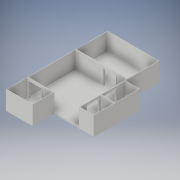
# Autodesk Inventor part: second floor down for landon
Saved by Autodesk Inventor 2017 (Build 210142000, 142)
## iProperties
Created: 2018-05-01
Part Number: second floor down for landon
Material: Generic
Document SubType Name: Modeling
Designer: braxtonwright
Density: 1 g/cm^3
Appearance: Default
Author: braxtonwright
Autodesk Inventor part; units mm, degrees
ref_plane "YZ Plane" through (0, 0, 0) normal (1, 0, 0) x (0, 1, 0)
ref_plane "XZ Plane" through (0, 0, 0) normal (0, 1, 0) x (-1, 0, 0)
ref_plane "XY Plane" through (0, 0, 0) normal (0, 0, 1) x (1, 0, 0)
sketch "Sketch1" plane through (0, 0, 0) normal (0, 1, 0) x (-1, 0, 0)
  line L0 (0, 0) -> (0, -901.7)
  line L1 (0, -901.7) -> (-774.7, -901.7) construction
  line L2 (-393.7, 0) -> (-520.7, 0)
  line L3 (0, 0) -> (0, 317.5)
  line L4 (0, 317.5) -> (-393.7, 317.5)
  line L5 (-393.7, 317.5) -> (-393.7, 0)
  line L6 (0, -901.7) -> (0, -1193.8)
  line L7 (0, -1193.8) -> (-774.7, -1193.8)
  line L8 (-774.7, -317.5) -> (-990.6, -317.5)
  line L9 (-990.6, -317.5) -> (-990.6, 0)
  line L10 (-990.6, 0) -> (-520.7, 0)
  line L11 (-990.6, -317.5) -> (-990.6, -685.8)
  line L12 (-990.6, -685.8) -> (-774.7, -685.8)
  line L13 (-393.7, 0) -> (0, 0) construction
  line L14 (-774.7, -1193.8) -> (-774.7, -901.7)
  line L15 (-774.7, -685.8) -> (-774.7, -901.7)
  dimension "d0" = 901.7
  dimension "d1" = 774.7
  dimension "d2" = 317.5
  dimension "d3" = 393.7
  dimension "d4" = 317.5
  dimension "d5" = 292.1
  dimension "d6" = 317.5
  dimension "d7" = 368.3
  dimension "d9" = 469.9
  dimension "d11" = 990.6
  dimension "d12" = 774.7
  constraints: 32 end point, 5 perpendicular, 4 vertical, 3 horizontal, 1 collinear
  measures "d0" distance of L0.start L0.end
  measures "d1" distance of L0.end L1.end
  measures "d2" distance of L0.start L3.end
  measures "d3" distance of L3.end L4.end
  measures "d4" distance between parallel lines of L2 L4
  measures "d5" distance of L0.end L6.end
  measures "d6" distance between parallel lines of L10 L8
  measures "d7" distance between parallel lines of L12 L8
  measures "d9" distance of L9.end L2.end
  measures "d11" distance between parallel lines of L0 L11
  measures "d12" distance from line of L8.start L0
extrude "floor" add sketch "Sketch1" along normal blind 25.4
sketch "Sketch2" plane through (0, 25.4, 0) normal (0, 1, 0) x (1, 0, 0)
  line L0 (0, 0) -> (0, 719.1204)
  line L1 (0, 719.1204) -> (774.7, 719.1204) construction
  line L2 (0, 0) -> (0, -317.5)
  line L3 (0, -317.5) -> (393.7, -317.5)
  line L4 (393.7, -317.5) -> (393.7, 0)
  line L5 (774.7, 317.5) -> (990.6, 317.5) construction
  line L6 (393.7, 0) -> (0, 0) construction
  line L7 (0, 1193.8) -> (0, -317.5) projected
  line L8 (393.7, 0) -> (990.6, 0) projected
  line L9 (774.7, 719.1204) -> (774.7, 317.5) construction
  line L10 (774.7, 317.5) -> (774.7, 0) construction
  line L11 (387.35, -311.15) -> (6.35, -311.15)
  line L12 (6.35, -311.15) -> (6.35, -6.35)
  line L13 (6.35, -6.35) -> (387.35, -6.35)
  line L14 (387.35, -6.35) -> (387.35, -311.15)
  line L15 (984.25, 679.45) -> (781.05, 679.45)
  line L16 (990.6, 685.8) -> (990.6, 0) projected
  line L17 (990.6, 685.8) -> (774.7, 685.8) projected
  line L18 (520.7, 685.8) -> (520.7, 1193.8) projected
  line L19 (774.7, 1193.8) -> (0, 1193.8) projected
  line L20 (768.35, 0) -> (990.6, 0)
  line L21 (990.6, 0) -> (990.6, 685.8)
  line L22 (990.6, 685.8) -> (774.7, 685.8)
  line L23 (774.7, 685.8) -> (774.7, 1193.8)
  line L24 (774.7, 1193.8) -> (0, 1193.8)
  line L25 (0, 1193.8) -> (0, 719.1204)
  line L26 (781.05, 6.35) -> (984.25, 6.35)
  line L27 (781.05, 311.15) -> (984.25, 311.15)
  line L28 (984.25, 323.85) -> (781.05, 323.85)
  line L29 (781.05, 6.35) -> (781.05, 311.15)
  line L30 (781.05, 323.85) -> (781.05, 679.45)
  line L31 (984.25, 6.35) -> (984.25, 311.15)
  line L32 (984.25, 323.85) -> (984.25, 679.45)
  line L33 (6.35, 6.35) -> (393.7, 6.35)
  line L34 (768.35, 1187.45) -> (6.35, 1187.45)
  line L35 (393.7, 0) -> (393.7, 6.35)
  line L36 (768.35, 6.35) -> (768.35, 0)
  line L37 (6.35, 725.4704) -> (768.35, 725.4704)
  line L38 (768.35, 712.7704) -> (6.35, 712.7704)
  line L39 (768.35, 6.35) -> (768.35, 712.7704)
  line L40 (768.35, 725.4704) -> (768.35, 1187.45)
  line L41 (6.35, 1187.45) -> (6.35, 725.4704)
  line L42 (6.35, 712.7704) -> (6.35, 6.35)
  line L43 (774.7, 685.8) -> (774.7, 1193.8) projected
  line L44 (393.7, -317.5) -> (393.7, 0) projected
  dimension "d27" = 317.5
  dimension "d28" = 6.35
  dimension "d34" = 6.35
  dimension "d39" = 6.35
  dimension "d40" = 6.35
  dimension "d41" = 6.35
  dimension "d42" = 6.35
  dimension "d43" = 6.35
  dimension "d48" = 6.35
  dimension "d50" = 6.35
  dimension "d63" = 12.7
  dimension "d64" = 6.35
  dimension "d67" = 984.25
  dimension "d68" = 0
  dimension "d69" = 679.45
  dimension "d114" = 6.35
  constraints: 74 end point, 14 perpendicular, 11 parallel, 8 collinear, 4 horizontal, 3 vertical, 2 point on line, 3 other
  measures "d27" distance between parallel lines of L5 L8
  measures "d28" distance between parallel lines of L3 L11
  measures "d34" distance between parallel lines of L17 L15
  measures "d39" distance between parallel lines of L26 L8
  measures "d40" distance between parallel lines of L5 L27
  measures "d41" distance between parallel lines of L28 L5
  measures "d42" distance between parallel lines of L16 L31
  measures "d43" horizontal distance of L5.start L27.start
  measures "d48" distance between parallel lines of L33 L8
  measures "d50" distance between parallel lines of L19 L34
  measures "d63" distance between parallel lines of L37 L38
  measures "d64" distance from line of L37.start L1
  measures "d67" distance between parallel lines of L16 L41
  measures "d68" distance from line of L5.end L16
  measures "d69" distance from line of L36.start L17
  measures "d114" distance between parallel lines of L39 L10
extrude "walls" add sketch "Sketch2" along normal blind 254 contours L0 L7 L19 L18 L34 L41 L37 L38 L42 L33 L35 L4 L3 L2 | L19 L23 L17 L16 L8 L36 L39 L38 L18 L37 L40 L34
sketch "Sketch4" plane through (0, 25.4, 0) normal (0, 1, 0) x (1, 0, 0)
  line L0 (387.35, -6.35) -> (6.35, -6.35) projected
  line L1 (387.35, -311.15) -> (387.35, -6.35) projected
  line L2 (6.35, -6.35) -> (387.35, -6.35)
  line L3 (387.35, -6.35) -> (387.35, -311.15)
  line L4 (6.35, -6.35) -> (6.35, -311.15) projected
  line L5 (387.35, -311.15) -> (6.35, -311.15)
  line L6 (6.35, -311.15) -> (6.35, -6.35)
  line L7 (6.35, -311.15) -> (387.35, -311.15) projected
  line L8 (6.35, -311.15) -> (387.35, -311.15)
  line L9 (8.4667, -8.4667) -> (385.2333, -8.4667)
  line L10 (385.2333, -8.4667) -> (385.2333, -309.0333)
  line L11 (385.2333, -309.0333) -> (8.4667, -309.0333)
  line L12 (8.4667, -309.0333) -> (8.4667, -8.4667)
  line L13 (781.05, 311.15) -> (781.05, 6.35) projected
  line L14 (984.25, 6.35) -> (984.25, 311.15) projected
  line L15 (781.05, 311.15) -> (984.25, 311.15)
  line L16 (984.25, 311.15) -> (984.25, 6.35)
  line L17 (984.25, 6.35) -> (781.05, 6.35)
  line L18 (781.05, 6.35) -> (781.05, 311.15)
  line L19 (781.05, 323.85) -> (781.05, 679.45) projected
  line L20 (984.25, 323.85) -> (781.05, 323.85) projected
  line L21 (781.05, 679.45) -> (984.25, 679.45)
  line L22 (984.25, 679.45) -> (984.25, 323.85)
  line L23 (984.25, 323.85) -> (781.05, 323.85)
  line L24 (781.05, 323.85) -> (781.05, 679.45)
  line L25 (982.1333, 677.3333) -> (783.1667, 677.3333)
  line L26 (783.1667, 677.3333) -> (783.1667, 325.9667)
  line L27 (783.1667, 325.9667) -> (982.1333, 325.9667)
  line L28 (982.1333, 325.9667) -> (982.1333, 677.3333)
  line L29 (982.1333, 309.0333) -> (783.1667, 309.0333)
  line L30 (783.1667, 309.0333) -> (783.1667, 8.4667)
  line L31 (783.1667, 8.4667) -> (982.1333, 8.4667)
  line L32 (982.1333, 8.4667) -> (982.1333, 309.0333)
  line L33 (768.35, 725.4704) -> (768.35, 1187.45) projected
  line L34 (768.35, 725.4704) -> (6.35, 725.4704) projected
  line L35 (768.35, 1187.45) -> (6.35, 1187.45)
  line L36 (6.35, 1187.45) -> (6.35, 725.4704)
  line L37 (6.35, 725.4704) -> (768.35, 725.4704)
  line L38 (768.35, 725.4704) -> (768.35, 1187.45)
  line L39 (8.4667, 1185.3333) -> (766.2333, 1185.3333)
  line L40 (766.2333, 1185.3333) -> (766.2333, 727.5871)
  line L41 (766.2333, 727.5871) -> (8.4667, 727.5871)
  line L42 (8.4667, 727.5871) -> (8.4667, 1185.3333)
  line L43 (768.35, 712.7704) -> (768.35, 0) projected
  line L44 (393.7, 6.35) -> (6.35, 6.35) projected
  line L45 (768.35, 712.7704) -> (6.35, 712.7704)
  line L46 (6.35, 712.7704) -> (6.35, 6.35)
  line L47 (768.35, 357.1704) -> (768.35, 712.7704)
  line L48 (766.2333, 710.6538) -> (8.4667, 710.6538)
  line L49 (8.4667, 710.6538) -> (8.4667, 8.4667)
  line L50 (8.4667, 8.4667) -> (395.8167, 8.4667)
  line L51 (766.2333, 359.2871) -> (766.2333, 710.6538)
  line L52 (393.7, 6.35) -> (393.7, 0) projected
  line L53 (393.7, 6.35) -> (393.7, 0)
  line L54 (393.7, 0) -> (395.8167, 0)
  line L55 (990.6, 0) -> (393.7, 0) projected
  line L56 (395.8167, 0) -> (395.8167, 8.4667)
  line L57 (768.35, 357.1704) -> (768.35, 0)
  line L58 (768.35, 0) -> (766.2333, 0)
  line L59 (766.2333, 359.2871) -> (766.2333, 0)
  line L60 (6.35, 6.35) -> (393.7, 6.35)
  line L61 (6.35, 1187.45) -> (768.35, 1187.45) projected
  dimension "d55" = 2.1167
  dimension "d56" = 2.1167
  dimension "d70" = 2.1167
  dimension "d76" = 2.1167
  dimension "d77" = 2.1167
  dimension "d78" = 2.1167
  dimension "d79" = 2.1167
  dimension "d80" = 2.1167
  constraints: 94 end point, 17 parallel, 12 perpendicular, 5 horizontal, 3 collinear, 3 point on line, 13 other
  measures "d55" distance between parallel lines of L21 L25
  measures "d56" distance between parallel lines of L15 L29
  measures "d70" distance between parallel lines of L0 L9
  measures "d76" distance between parallel lines of L35 L39
  measures "d77" distance between parallel lines of L47 L51
  measures "d78" distance of L53.end L54.end
  measures "d79" distance between parallel lines of L44 L50
  measures "d80" distance between parallel lines of L46 L49
extrude "trim" add sketch "Sketch4" along normal blind 21.0312 contours L1 L5 L4 L0 | L15 L14 L17 L13 | L19 L21 L22 L20 | L34 L36 L35 L33 | L43 L55 L59 L51 L48 L49 L50 L56 L54 L52 L44 L46 L45
sketch "Sketch5" plane through (783.1667, 25.4, -8.4667) normal (1, 0, 0) x (0, 0, -1)
  line L0 (0, 0) -> (300.5667, 0) projected
  line L1 (277.2833, 0) -> (86.7833, 0)
  line L2 (86.7833, 0) -> (86.7833, 223.52)
  line L3 (86.7833, 223.52) -> (277.2833, 223.52)
  line L4 (277.2833, 223.52) -> (277.2833, 0)
  line L5 (302.6833, 21.0312) -> (302.6833, 254) projected
  line L6 (315.3833, 21.0312) -> (315.3833, 254) projected
  line L7 (315.3833, 254) -> (302.6833, 254)
  line L8 (-8.4667, 254) -> (677.3333, 254) projected
  line L9 (309.0333, 254) -> (309.0333, -25.4) construction
  line L10 (340.7833, 0) -> (531.2833, 0)
  line L11 (531.2833, 0) -> (531.2833, 223.52)
  line L12 (531.2833, 223.52) -> (340.7833, 223.52)
  line L13 (340.7833, 223.52) -> (340.7833, 0)
  point P0 (-8.4667, -25.4)
  dimension "d59" = 190.5
  dimension "d60" = 223.52
  dimension "d61" = 25.4
  constraints: 20 end point, 4 symmetric about line, 2 parallel, 1 collinear, 1 horizontal, 1 midpoint, 1 perpendicular, 1 point on line, 1 vertical
  measures "d59" distance of L2.end L3.end
  measures "d60" distance of L1.end L2.end
  measures "d61" distance between parallel lines of L5 L4
extrude "doorframe 1 and 2" cut sketch "Sketch5" against normal up to surface (14.8167 mm away)
sketch "Sketch6" plane through (766.2333, 25.4, -727.5871) normal (0, 0, -1) x (-1, 0, 0)
  line L0 (150.2833, 223.52) -> (340.7833, 223.52)
  line L1 (340.7833, 223.52) -> (340.7833, 0)
  line L2 (340.7833, 0) -> (150.2833, 0)
  line L3 (150.2833, 0) -> (150.2833, 223.52)
  line L4 (-8.4667, 7.9325) -> (-8.4667, 240.144)
  line L5 (-8.4667, -25.4) -> (-8.4667, 254) projected
  line L6 (0, 0) -> (757.7667, 0) projected
  point P0 (503.7667, 0)
  point P1 (245.5333, 223.52)
  dimension "d83" = 190.5
  dimension "d84" = 223.52
  dimension "d86" = 254
  constraints: 10 end point, 2 collinear, 2 parallel, 1 horizontal, 1 midpoint, 1 perpendicular, 1 vertical
  measures "d83" distance of L1.end L2.end
  measures "d84" distance of L0.end L1.end
  measures "d86" distance from line of L4 point (245.533, 223.52)
extrude "door frame 3" cut sketch "Sketch6" against normal up to surface (16.9333 mm away)
sketch "Sketch7" plane through (395.8167, 25.4, -8.4667) normal (0, 0, -1) x (-1, 0, 0)
  line L0 (173.5667, 223.52) -> (364.0667, 223.52)
  line L1 (364.0667, 223.52) -> (364.0667, 0)
  line L2 (364.0667, 0) -> (173.5667, 0)
  line L3 (173.5667, 0) -> (173.5667, 223.52)
  line L4 (10.5833, 0) -> (387.35, 0) projected
  line L5 (389.4667, 21.0312) -> (389.4667, 254) projected
  point P0 (395.8167, -25.4)
  dimension "d89" = 190.5
  dimension "d90" = 223.52
  dimension "d91" = 25.4
  constraints: 8 end point, 2 parallel, 1 collinear, 1 horizontal, 1 perpendicular
  measures "d89" distance of L1.end L2.end
  measures "d90" distance of L0.end L1.end
  measures "d91" distance between parallel lines of L5 L1
extrude "door frame 4" cut sketch "Sketch7" against normal up to surface (16.9333 mm away)
ref_plane "door trim workplane 1 and 2" through (774.7, 279.4, -6.35) normal (1, 0, 0) x (0, 0, -1)
sketch "Sketch8" plane through (774.7, 279.4, -6.35) normal (1, 0, 0) x (0, 0, -1)
  line L0 (342.9, -30.48) -> (533.4, -30.48) projected
  line L1 (670.9833, -254) -> (319.6167, -254) projected
  line L2 (533.4, -30.48) -> (342.9, -30.48)
  line L3 (342.9, -30.48) -> (342.9, -254)
  line L4 (533.4, -254) -> (533.4, -30.48)
  line L5 (88.9, -254) -> (88.9, -232.9688) projected
  line L6 (279.4, -30.48) -> (88.9, -30.48)
  line L7 (88.9, -30.48) -> (88.9, -254)
  line L8 (279.4, -254) -> (279.4, -30.48)
  line L9 (541.147, -22.733) -> (335.153, -22.733)
  line L10 (335.153, -22.733) -> (335.153, -254)
  line L11 (541.147, -254) -> (541.147, -22.733)
  line L12 (81.153, -22.733) -> (287.147, -22.733)
  line L13 (287.147, -22.733) -> (287.147, -254)
  line L14 (81.153, -254) -> (81.153, -22.733)
  line L15 (319.6167, -254) -> (670.9833, -254) projected
  line L16 (541.147, -254) -> (533.4, -254)
  line L17 (342.9, -254) -> (335.153, -254)
  line L18 (2.1167, -254) -> (302.6833, -254) projected
  line L19 (287.147, -254) -> (279.4, -254)
  line L20 (88.9, -254) -> (81.153, -254)
  point P0 (-6.35, -279.4)
  dimension "d94" = 7.747
  dimension "d95" = 7.747
  dimension "d96" = 7.747
  dimension "d97" = 7.747
  dimension "d98" = 7.747
  dimension "d99" = 7.747
  constraints: 32 end point, 4 parallel, 4 perpendicular, 4 point on line, 2 collinear, 2 horizontal
  measures "d94" distance between parallel lines of L4 L11
  measures "d95" distance between parallel lines of L6 L12
  measures "d96" distance between parallel lines of L0 L9
  measures "d97" distance between parallel lines of L10 L3
  measures "d98" distance between parallel lines of L8 L13
  measures "d99" distance between parallel lines of L14 L7
extrude "door trim 1 and 2" add sketch "Sketch8" along normal mid plane 25.4 contours L3 L1 L10 L9 L11 L4 L0 | L18 L14 L12 L13 L8 L6 L7 L5
ref_plane "door time workplane 3" through (6.35, 279.4, -719.1204) normal (0, 0, 1) x (1, 0, 0)
sketch "Sketch9" plane through (6.35, 279.4, -719.1204) normal (0, 0, 1) x (1, 0, 0)
  line L0 (609.6, -30.48) -> (419.1, -30.48)
  line L1 (419.1, -30.48) -> (419.1, -254)
  line L2 (609.6, -254) -> (609.6, -30.48)
  line L3 (411.353, -22.733) -> (617.347, -22.733)
  line L4 (617.347, -22.733) -> (617.347, -254)
  line L5 (411.353, -254) -> (411.353, -22.733)
  line L6 (617.347, -254) -> (609.6, -254)
  line L7 (419.1, -254) -> (411.353, -254)
  line L8 (609.6, -232.9688) -> (609.6, -30.48) projected
  line L9 (609.6, -30.48) -> (419.1, -30.48) projected
  line L10 (419.1, -30.48) -> (419.1, -232.9688) projected
  line L11 (759.8833, -254) -> (2.1167, -254) projected
  point P0 (-6.35, -279.4)
  point P1 (-6.35, -279.4)
  dimension "d102" = 7.747
  dimension "d103" = 7.747
  dimension "d104" = 7.747
  constraints: 16 end point, 5 collinear, 3 perpendicular, 2 parallel, 1 horizontal, 1 point on line
  measures "d102" distance between parallel lines of L0 L3
  measures "d103" distance between parallel lines of L2 L4
  measures "d104" distance between parallel lines of L5 L1
extrude "door trim 3" add sketch "Sketch9" along normal mid plane 25.4 contours L0 L1 L7 L5 L3 L4 L6 L2
ref_plane "Work Plane3" through (395.8167, 25.4, 0) normal (0, 0, -1) x (-1, 0, 0)
sketch "Sketch10" plane through (395.8167, 25.4, 0) normal (0, 0, -1) x (-1, 0, 0)
  line L0 (371.8137, 231.267) -> (371.8137, 0)
  line L1 (364.0667, 0) -> (364.0667, 223.52)
  line L2 (371.8137, 0) -> (364.0667, 0)
  line L3 (173.5667, 0) -> (165.8197, 0)
  line L4 (364.0667, 223.52) -> (173.5667, 223.52)
  line L5 (173.5667, 223.52) -> (173.5667, 0)
  line L6 (165.8197, 231.267) -> (371.8137, 231.267)
  line L7 (165.8197, 0) -> (165.8197, 231.267)
  line L8 (364.0667, 223.52) -> (364.0667, 22.2122)
  line L9 (364.0667, 21.0312) -> (364.0667, 0) projected
  line L10 (173.5667, 21.0312) -> (173.5667, 223.52) projected
  line L11 (173.5667, 0) -> (173.5667, 21.0312) projected
  line L12 (173.5667, 223.52) -> (364.0667, 223.52) projected
  point P0 (395.8167, -25.4)
  dimension "d108" = 7.747
  dimension "d109" = 7.747
  dimension "d110" = 7.747
  constraints: 18 end point, 3 perpendicular, 2 parallel, 1 collinear, 1 horizontal, 1 point on line
  measures "d108" distance between parallel lines of L4 L6
  measures "d109" distance between parallel lines of L1 L0
  measures "d110" distance between parallel lines of L7 L5
extrude "door trim 4" add sketch "Sketch10" along normal mid plane 25.4
equation "\"d34\" = d28"
equation "\"d39\" = d28"
equation "\"d40\" = d28"
equation "\"d41\" = d28"
equation "\"d42\" = d28"
equation "\"d43\" = d28"
equation "\"d48\" = d28"
equation "\"d50\" = d28"
equation "\"d63\" = 2 * d28"
equation "\"d64\" = d28"
equation "\"d55\" = d52"
equation "\"d56\" = d52"
equation "\"d70\" = d52"
equation "\"d76\" = d52"
equation "\"d77\" = d52"
equation "\"d78\" = d52"
equation "\"d79\" = d52"
equation "\"d80\" = d52"
equation "\"d95\" = d94"
equation "\"d96\" = d94"
equation "\"d97\" = d94"
equation "\"d98\" = d94"
equation "\"d99\" = d94"
equation "\"d102\" = d105"
equation "\"d103\" = d105"
equation "\"d104\" = d105"
equation "\"d108\" = d111"
equation "\"d109\" = d111"
equation "\"d110\" = d111"
equation "\"d30\" = d28"
equation "\"d31\" = d28"
equation "\"d38\" = d28"
equation "\"d49\" = d28"
equation "\"d51\" = d28"
equation "\"d71\" = d52"
equation "\"d52\" = 2.116667"
equation "\"d105\" = 7.747"
equation "\"d111\" = 7.747"
body "Solid1"
